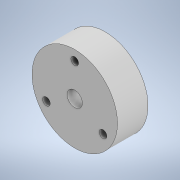
# Autodesk Inventor part: Burner Table IS v01
Saved by Autodesk Inventor 2020 (Build 240168000, 168)
## iProperties
Created: 2019-06-07
Part Number: Burner Table IS v01
Material: Generic
Document SubType Name: Modeling
Designer: isadmin
Density: 1 g/cm^3
Appearance: Default
Author: isadmin
Autodesk Inventor part; units mm, degrees
ref_plane "YZ Plane" through (0, 0, 0) normal (1, 0, 0) x (0, 1, 0)
ref_plane "XZ Plane" through (0, 0, 0) normal (0, 1, 0) x (-1, 0, 0)
ref_plane "XY Plane" through (0, 0, 0) normal (0, 0, 1) x (1, 0, 0)
sketch "Sketch1" plane through (0, 0, 0) normal (0, 0, 1) x (1, 0, 0)
  circle A0 centre (0, 0) radius 17.78
  circle A1 centre (0, 0) radius 3.175
  circle A2 centre (0, 0) radius 13.6153
  circle A3 centre (0, 13.6153) radius 1.5875
  circle A4 centre (-11.7912, -6.8077) radius 1.5875
  circle A5 centre (11.7912, -6.8077) radius 1.5875
  dimension "d2" = 27.2307
  dimension "d0" = 35.56
  dimension "d1" = 6.35
  dimension "d3" = 3.175
  dimension "d6" = 360
  constraints: 5 centre point, 3 coincident, 1 vertical alignment, 12 other
  measures "d0" diameter of A0
  measures "d1" diameter of A1
  measures "d3" diameter of A3
extrude "Extrusion1" add sketch "Sketch1" along normal blind 12.7 contours A0 | A2 A5 A4 A3
body "Solid1"
